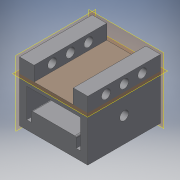
# Autodesk Inventor part: NASA Objektträgerhalter (Südkorea)
Saved by Autodesk Inventor 2018.3 (Build 223284000, 284)
## iProperties
Created: 2018-04-26
Part Number: NASA Objektträgerhalter (Südkorea)
Material: Allgemein
Document SubType Name: Modeling
Designer: pgmadmin
Density: 1 g/cm^3
Appearance: Vorgabe
Author: pgmadmin
Autodesk Inventor part; units mm, degrees
sketch "Skizze1" plane through (0, 0, 0) normal (0, 0, 1) x (1, 0, 0)
  line L0 (-9.4, 0) -> (56.4, 0) projected
  line L1 (0, -37.2) -> (0, 6.2) projected
  line L2 (0, 0) -> (47, 0)
  line L3 (47, 0) -> (47, -31)
  line L4 (47, -31) -> (0, -31)
  line L5 (0, -31) -> (0, 0)
  line L6 (5, -5) -> (42, -5)
  line L7 (42, -5) -> (42, -25)
  line L8 (42, -25) -> (39, -25)
  line L9 (39, -25) -> (39, -18)
  line L10 (39, -18) -> (8, -18)
  line L11 (8, -18) -> (8, -25)
  line L12 (8, -25) -> (5, -25)
  line L13 (5, -25) -> (5, -5)
  dimension "d0" = 47
  dimension "d1" = 31
  dimension "d2" = 5
  dimension "d3" = 5
  dimension "d4" = 5
  dimension "d5" = 6
  dimension "d6" = 6
  dimension "d7" = 3
  dimension "d8" = 3
  dimension "d9" = 13
  constraints: 24 end point, 8 perpendicular, 2 horizontal, 2 parallel
  measures "d0" distance of L3.end L4.end
  measures "d1" distance of L2.end L3.end
  measures "d2" distance between parallel lines of L2 L6
  measures "d3" distance between parallel lines of L3 L7
  measures "d4" distance between parallel lines of L5 L13
  measures "d5" distance between parallel lines of L4 L12
  measures "d6" distance between parallel lines of L4 L8
  measures "d7" distance between parallel lines of L7 L9
  measures "d8" distance between parallel lines of L13 L11
  measures "d9" distance between parallel lines of L10 L6
extrude "Extrusion1" add sketch "Skizze1" along normal blind 50
fillet "Rundung1" radius 1 2 edges at (8, -18, 25) (39, -18, 25)
sketch "Skizze4" plane through (0, -31, 0) normal (-1, 0, 0) x (0, 0, 1)
  line L0 (50, 31) -> (50, 0) projected
  line L1 (0, 31) -> (50, 31) projected
  circle A0 centre (25, 17) radius 1.8
  dimension "d41" = 25
  dimension "d42" = 14
  dimension "d43" = 3.6
  constraints: 1 centre point, 1 coincident
  measures "d41" distance from line of L0 point (25, 17)
  measures "d42" distance from line of point (25, 17) L1
  measures "d43" diameter of A0
hole "Bohrung3" at (0, -14, 25) direction (1, 0, 0) diameter 6.15 end through all
sketch "Skizze5" plane through (0, 0, 0) normal (0, 1, 0) x (1, 0, 0)
  line L0 (0, 0) -> (47, 0) projected
  line L1 (0, 0) -> (10, 0)
  line L2 (10, 0) -> (10, -50)
  line L3 (10, -50) -> (0, -50)
  line L4 (0, -50) -> (0, 0)
  line L5 (47, 0) -> (47, -50) projected
  line L6 (47, 0) -> (37, 0)
  line L7 (37, 0) -> (37, -50)
  line L8 (37, -50) -> (47, -50)
  line L9 (47, -50) -> (47, 0)
  dimension "d51" = 10
  dimension "d52" = 50
  dimension "d53" = 10
  dimension "d54" = 50
  constraints: 16 end point, 4 parallel, 2 horizontal, 2 perpendicular
  measures "d51" distance of L2.end L3.end
  measures "d52" distance of L1.end L2.end
  measures "d53" distance of L8.end L7.end
  measures "d54" distance of L7.end L6.end
extrude "Extrusion4" add sketch "Skizze5" along normal blind 10
sketch "Skizze6" plane through (47, -31, 50) normal (1, 0, 0) x (0, 0, -1)
  line L0 (0, 41) -> (50, 41) projected
  line L1 (50, 41) -> (50, 0) projected
  line L2 (0, 0) -> (0, 41) projected
  point P0 (50, 31)
  point P1 (12.5, 36)
  point P2 (25, 36)
  point P3 (37.5, 36)
  dimension "d57" = 5
  dimension "d58" = 5
  dimension "d59" = 5
  dimension "d60" = 12.5
  dimension "d61" = 12.5
  dimension "d62" = 12.5
  measures "d57" distance from line of L0 point (25, 36)
  measures "d58" distance from line of L0 point (12.5, 36)
  measures "d59" distance from line of L0 point (37.5, 36)
  measures "d60" distance from line of L1 point (37.5, 36)
  measures "d61" distance from line of L2 point (12.5, 36)
  measures "d62" distance of point (12.5, 36) point (25, 36)
hole "Bohrung4" at (47, 5, 37.5) at (47, 5, 25) at (47, 5, 12.5) direction (-1, 0, 0) diameter 6.15 end through all
